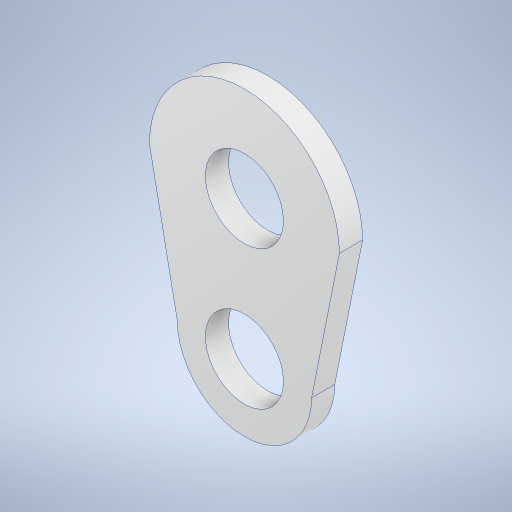
# Autodesk Inventor part: Bottom Plate
Saved by Autodesk Inventor 2024.4 (Build 284460000, 460)
## iProperties
Created: 2026-06-13
Part Number: Bottom Plate
Material: Aluminum 6061
Document SubType Name: Modeling
Designer: stanc
Density: 2.7 g/cm^3
Appearance: Aluminum - Flat
Author: stanc
Autodesk Inventor part; units mm, degrees
ref_plane "YZ Plane" through (0, 0, 0) normal (1, 0, 0) x (0, 1, 0)
ref_plane "XZ Plane" through (0, 0, 0) normal (0, 1, 0) x (-1, 0, 0)
ref_plane "XY Plane" through (0, 0, 0) normal (0, 0, 1) x (1, 0, 0)
sketch "Sketch1" plane through (0, 0, 0) normal (0, 0, 1) x (1, 0, 0)
  circle A0 centre (0, 0) radius 15.24
  circle A1 centre (0, 0) radius 10.7061
  circle A2 centre (0, 38.1) radius 22.86
  line L0 (0, 15.24) -> (0, 16.764)
  circle A3 centre (0, 38.1) radius 26.035
  circle A4 centre (0, 0) radius 18.415
  circle A5 centre (0, 38.1) radius 10.7061
  line L1 (0, 15.24) -> (0, 15.24)
  line L2 (-18.415, 0) -> (-26.035, 38.1)
  line L3 (18.415, 0) -> (26.035, 38.1)
  arc A6 (26.035, 38.1) -> (-26.035, 38.1) centre (0, 38.1) ccw
  arc A7 (-18.415, 0) -> (18.415, 0) centre (0, 0) ccw
  dimension "d0" = 30.48
  dimension "d3" = 45.72
  dimension "d1" = 21.4122
  dimension "d4" = 52.07
  dimension "d5" = 36.83
  dimension "d6" = 21.4122
  constraints: 8 end point, 8 point on circle, 6 centre point, 6 coincident, 4 concentric, 2 vertical, 2 vertical alignment, 4 other
  measures "d1" diameter of A1
  measures "d4" diameter of A3
  measures "d5" diameter of A4
  measures "d6" diameter of A5
extrude "Extrusion1" add sketch "Sketch1" along normal blind 6.35 contours A0 A3 | A0 A3 A4 | A3 A0 | A0 A2 A4 A3 | A3 A4 A2 A0 | A2 A4 | A4 A2 A3 L2 L3 | A3 L3 A4 | A4 L2 A3 | A2 A4
body "Solid1"
